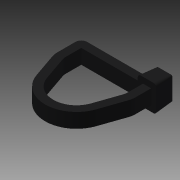
# Autodesk Inventor part: fastener_01
Saved by Autodesk Inventor 2013 (Build 170138000, 138)
## iProperties
Shininess: 41.0
Created: 2014-03-04
Part Number: fastener_01
Document SubType Name: Modeling
Designer: Noa Izumi
Material: Default
Density: 1 g/cm^3
Density: 0.0
Volumn: 0.0
Area: 0.0
PropertySet Name: Model Information
Control State: 0
Master: False
Checked Out: False
Author: Noa Izumi
Autodesk Inventor part; units mm, degrees
ref_plane "YZ Plane" through (0, 0, 0) normal (1, 0, 0) x (0, 1, 0)
ref_plane "XZ Plane" through (0, 0, 0) normal (0, 1, 0) x (-1, 0, 0)
ref_plane "XY Plane" through (0, 0, 0) normal (0, 0, 1) x (1, 0, 0)
sketch "Sketch1" plane through (0, 0, 0) normal (0, 0, 1) x (1, 0, 0)
  arc A0 (3.1723, -7.3022) -> (10.7365, -7.3022) centre (6.9544, -6) ccw
  line L0 (1.6544, 0.1064) -> (1.6544, -2.5589)
  line L1 (1.6544, 0.1064) -> (12.2544, 0.1064)
  line L2 (12.2544, 0.1064) -> (12.2544, -2.5589)
  line L3 (1.7634, -3.21) -> (3.1723, -7.3022)
  line L4 (12.1455, -3.21) -> (10.7365, -7.3022)
  arc A1 (1.6544, -2.5589) -> (1.7634, -3.21) centre (3.6544, -2.5589) ccw
  arc A2 (12.1455, -3.21) -> (12.2544, -2.5589) centre (10.2544, -2.5589) ccw
  line L5 (12.0603, -7.7579) -> (13.4692, -3.6658)
  arc A3 (13.4692, -3.6658) -> (13.6544, -2.5589) centre (10.2544, -2.5589) ccw
  line L6 (13.6544, -2.5589) -> (13.6544, 1.5064)
  line L7 (13.6544, 1.5064) -> (1.2544, 1.5064)
  line L8 (0.2544, 0.5064) -> (0.2544, -2.5589)
  arc A4 (0.2544, -2.5589) -> (0.4396, -3.6658) centre (3.6544, -2.5589) ccw
  line L9 (0.4396, -3.6658) -> (1.8486, -7.7579)
  arc A5 (1.8486, -7.7579) -> (12.0603, -7.7579) centre (6.9544, -6) ccw
  arc A6 (1.2544, 1.5064) -> (0.2544, 0.5064) centre (1.2544, 0.5064) ccw
  point P0 (1.6544, -2.8936)
  point P1 (12.2544, -2.8936)
  point P2 (13.6544, 0.2)
  point P3 (12.7544, 1.5064)
  dimension "d12" = 4
  dimension "d13" = 3
  dimension "d14" = 3
  dimension "d16" = 2
  dimension "d17" = 1.4
  dimension "d18" = 1
  dimension "d35" = 10.6
  constraints: 20 end point, 14 point on circle, 14 tangent, 7 centre point, 6 point on line, 2 parallel, 1 equal radius, 1 horizontal, 1 vertical, 4 other
  measures "d12" radius of A0
  measures "d13" distance of L1.end point (12.254, -2.894)
  measures "d14" distance of L0.start point (1.654, -2.894)
  measures "d16" radius of A1
  measures "d17" distance between parallel lines of L5 L4
  measures "d18" radius of A6
  measures "d35" distance between parallel lines of L2 L0
extrude "Extrusion1" add sketch "Sketch1" along normal blind 2.5
sketch "Sketch3" plane through (1.6544, 0.1064, 2.5) normal (0, -1, 0) x (1, 0, 0)
  line L0 (10.2, 1) -> (12.4, 1)
  line L1 (12.9, 0.5) -> (12.9, -3)
  line L2 (12.4, -3.5) -> (10.2, -3.5)
  line L3 (9.7, -3) -> (9.7, 0.5)
  arc A0 (12.9, 0.5) -> (12.4, 1) centre (12.4, 0.5) ccw
  arc A1 (12.4, -3.5) -> (12.9, -3) centre (12.4, -3) ccw
  arc A2 (9.7, -3) -> (10.2, -3.5) centre (10.2, -3) ccw
  arc A3 (10.2, 1) -> (9.7, 0.5) centre (10.2, 0.5) ccw
  line L4 (-1.4, -2.5) -> (-1.4, 0) projected
  point P0 (9.7, 1)
  point P1 (12.9, -3.5)
  point P2 (12.9, 1)
  point P3 (9.7, -3.5)
  dimension "d21" = 4.5
  dimension "d22" = 3.2
  dimension "d27" = 0.5
  dimension "d36" = 11.1
  constraints: 8 end point, 8 point on circle, 8 point on line, 8 tangent, 4 centre point, 3 equal radius, 2 parallel, 1 horizontal, 1 perpendicular
  measures "d21" distance of point (9.7, -3.5) point (9.7, 1)
  measures "d22" distance of point (9.7, 1) point (12.9, 1)
  measures "d27" radius of A0
  measures "d36" distance between parallel lines of L4 L3
extrude "Extrusion2" add sketch "Sketch3" against normal blind 3 draft -5
